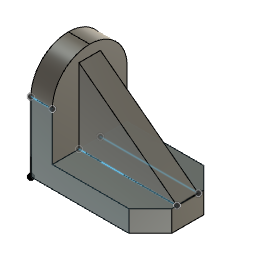
A1 (Autodesk Fusion 360 design; units mm, degrees)
Autodesk Fusion 360 part; units mm, degrees
sketch "Sketch1" plane through (0, 0, 0) normal (0, 0, 1) x (1, 0, 0)
  line L0 (0, 0) -> (55, 0)
  line L1 (67, 12) -> (67, 30)
  line L2 (55, 42) -> (0, 42)
  line L3 (0, 42) -> (0, 0)
  line L4 (67, 0) -> (55, 0) construction
  line L5 (55, 0) -> (55, 12) construction
  line L6 (55, 12) -> (67, 12) construction
  line L7 (67, 12) -> (67, 0) construction
  line L8 (67, 42) -> (55, 42) construction
  line L9 (55, 42) -> (55, 30) construction
  line L10 (55, 30) -> (67, 30) construction
  line L11 (67, 30) -> (67, 42) construction
  line L12 (55, 0) -> (67, 12)
  line L13 (55, 42) -> (67, 30)
  line L14 (0, 42) -> (13, 42)
  line L15 (13, 42) -> (13, 0)
  line L16 (13, 0) -> (0, 0)
  line L17 (0, 0) -> (0, 42)
  line L18 (13, 21) -> (67, 21)
  line L19 (67, 21) -> (13, 21)
  line L20 (13, 27) -> (67, 27)
  line L21 (67, 27) -> (67, 21)
  line L22 (13, 15) -> (67, 15)
  constraint horizontal L0
  constraint vertical L1
  constraint horizontal L2
  constraint vertical L3
  constraint coincident L0.start L3.end
  constraint horizontal L4
  constraint vertical L5
  constraint horizontal L6
  constraint vertical L7
  constraint horizontal L8
  constraint vertical L9
  constraint horizontal L10
  constraint vertical L11
  constraint perpendicular L12 L13
  constraint horizontal L14
  constraint vertical L15
  constraint horizontal L16
  constraint vertical L17
  constraint coincident L0 L15.end
  constraint midpoint L15 L18.start
  constraint midpoint L1 L18.end
  constraint perpendicular L1 L18
  constraint horizontal L19
  constraint horizontal L20
  constraint vertical L21
  constraint coincident L15 L20.start
  constraint symmetric L18 L20.end L22.end
  constraint symmetric L18 L20.start L22.start
extrude "Extrude1" add sketch "Sketch1" along normal blind 12
sketch "Sketch4" plane through (0, 0, 12) normal (0, 0, 1) x (-1, 0, 0)
  line L0 (-55, -42) -> (0, -42)
  line L1 (0, -42) -> (0, 0)
  line L2 (0, 0) -> (-55, 0)
  line L3 (-55, 0) -> (-67, -12)
  line L4 (-67, -12) -> (-67, -30)
  line L5 (-67, -30) -> (-55, -42)
  line L6 (0, -42) -> (-12, -42)
  line L7 (-12, -42) -> (-12, 0)
  line L8 (-12, 0) -> (0, 0)
  line L9 (0, 0) -> (0, -42)
  constraint horizontal L6
  constraint vertical L7
  constraint horizontal L8
  constraint vertical L9
  constraint coincident L2 L7.end
  constraint coincident L0.end L1.start
extrude "Extrude2" add sketch "Sketch4" along normal blind 27 contours L0 L1 L2 L6 L7 L8 L9
sketch "Sketch5" plane through (0, 0, 39) normal (0, 0, 1) x (-1, 0, 0)
  line L0 (0, 0) -> (-12, 0)
  line L1 (-12, 0) -> (-12, -42)
  line L2 (-12, -42) -> (0, -42)
  line L3 (0, -42) -> (0, 0)
  line L4 (0, -42) -> (-12, -42)
  line L5 (-12, -42) -> (-12, 0)
  line L6 (-12, 0) -> (0, 0)
  line L7 (0, 0) -> (0, -42)
  constraint horizontal L4
  constraint vertical L5
  constraint horizontal L6
  constraint vertical L7
  constraint coincident L0.end L1.start
  constraint coincident L2.end L3.start
extrude "Extrude3" add sketch "Sketch5" along normal blind 21
fillet "Fillet1" radius 21 1 edges at (6, 0, 60)
sketch "Sketch6" plane through (0, 0, 0) normal (0, -1, 0) x (1, 0, 0)
  line L0 (12, 39) -> (0, 39)
  line L1 (0, 39) -> (0, 0)
  line L2 (0, 0) -> (55, 0)
  line L3 (55, 0) -> (55, 12)
  line L4 (55, 12) -> (12, 12)
  line L5 (12, 12) -> (12, 39)
  line L6 (0, 0) -> (0, 39)
  line L7 (0, 39) -> (12, 39)
  constraint coincident L1.end L2.start
  constraint coincident L1 L0.end
  constraint perpendicular L0 L6
  constraint coincident L5 L0.start
  constraint perpendicular L5 L7
fillet "Fillet2" radius 21 1 edges at (6, 42, 60)
sketch "Sketch7" plane through (0, 0, 12) normal (0, 0, 1) x (-1, 0, 0)
  line L0 (-12, -42) -> (-12, 0)
  line L1 (-12, 0) -> (-55, 0)
  line L2 (-55, 0) -> (-67, -12)
  line L3 (-67, -12) -> (-67, -30)
  line L4 (-67, -30) -> (-55, -42)
  line L5 (-55, -42) -> (-12, -42)
  line L6 (-25, -15) -> (-12, -15)
  line L7 (-25, -15) -> (-67, -15)
  line L8 (-67, -15) -> (-67, -27)
  line L9 (-67, -27) -> (-12, -27)
  constraint coincident L0 L6.end
  constraint perpendicular L0 L6
  constraint coincident L3 L7.end
  constraint perpendicular L3 L7
  constraint coincident L3 L8.end
  constraint coincident L0 L9.end
  constraint perpendicular L0 L9
sketch "Sketch8" plane through (0, 0, 0) normal (0, -1, 0) x (1, 0, 0)
  line L0 (12, 12) -> (12, 54)
  line L1 (12, 54) -> (67, 12)
  line L2 (12, 12) -> (67, 12)
  constraint vertical L0
  constraint perpendicular L0 L2
extrude "Extrude4" add sketch "Sketch8" against normal blind 27
sketch "Sketch9" plane through (0, 0, 0) normal (0, -1, 0) x (1, 0, 0)
  line L0 (12, 39) -> (0, 39)
  line L1 (0, 39) -> (0, 0)
  line L2 (0, 0) -> (55, 0)
  line L3 (55, 0) -> (55, 12)
  line L4 (55, 12) -> (67, 12)
  line L5 (67, 12) -> (12, 54)
  line L6 (12, 54) -> (12, 39)
  line L7 (12, 54) -> (12, 12)
  line L8 (12, 12) -> (67, 12)
  line L9 (12, 54) -> (67, 12)
  constraint coincident L5.end L6.start
  constraint parallel L6 L7
  constraint coincident L4.end L5.start
  constraint perpendicular L7 L8
extrude "Extrude5" cut sketch "Sketch9" against normal blind 15 contours L4 L5 L6 L7 L8 L9
